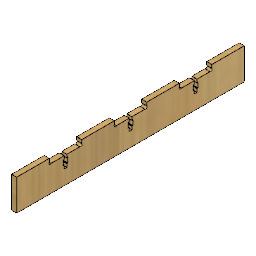
Bottom-plate-IIIS-square-rev1-40mm_8mm v1 (Autodesk Fusion 360 design; units mm, degrees)
Autodesk Fusion 360 part; units mm, degrees
sketch "Basic shape" plane through (0, 0, 0) normal (1, 0, 0) x (0, 0, -1)
  line L0 (0, 0) -> (-348.5, 0)
  line L1 (-348.5, 0) -> (-348.5, -48)
  line L2 (-348.5, -48) -> (0, -48)
  line L3 (0, -48) -> (0, 0)
  line L4 (-50, 0) -> (-99.5, 0)
  line L5 (-99.5, 0) -> (-99.5, -8)
  line L6 (-99.5, -8) -> (-50, -8)
  line L7 (-50, -8) -> (-50, 0)
  line L8 (-149.5, 0) -> (-199, 0)
  line L9 (-199, 0) -> (-199, -8)
  line L10 (-199, -8) -> (-149.5, -8)
  line L11 (-149.5, -8) -> (-149.5, 0)
  line L12 (-249, 0) -> (-298.5, 0)
  line L13 (-298.5, 0) -> (-298.5, -8)
  line L14 (-298.5, -8) -> (-249, -8)
  line L15 (-249, -8) -> (-249, 0)
  line L16 (-298.5, -8) -> (-348.5, -8) construction
  line L17 (-199, -8) -> (-249, -8) construction
  line L18 (-99.5, -8) -> (-149.5, -8) construction
  line L19 (-50, -8) -> (0, -8) construction
  dimension "d10" = 50
  dimension "d12" = 8
  dimension "d13" = 348.5
  dimension "d14" = 36.1667
  dimension "d246" = 40
  measures "d13" distance of L0.start
extrude "Extrude1" add sketch "Basic shape" along normal blind 8 contours L0 L1 L2 L3 L5 L6 L7 L9 L10 L11 L13 L14 L15
sketch "T slots" plane through (0, 0, 0) normal (-1, 0, 0) x (0, 0, 1)
  line L0 (348.5, 0) -> (298.5, 0)
  line L1 (298.5, 0) -> (298.5, -8)
  line L2 (298.5, -8) -> (249, -8)
  line L3 (249, -8) -> (249, 0)
  line L4 (249, 0) -> (199, 0)
  line L5 (199, 0) -> (199, -8)
  line L6 (199, -8) -> (149.5, -8)
  line L7 (149.5, -8) -> (149.5, 0)
  line L8 (149.5, 0) -> (99.5, 0)
  line L9 (99.5, 0) -> (99.5, -8)
  line L10 (99.5, -8) -> (50, -8)
  line L11 (50, -8) -> (50, 0)
  line L12 (50, 0) -> (0, 0)
  line L13 (0, 0) -> (0, -48)
  line L14 (0, -48) -> (348.5, -48)
  line L15 (348.5, -48) -> (348.5, 0)
  line L16 (72.74, -8) -> (76.76, -8)
  line L17 (76.76, -8) -> (76.76, -25.5)
  line L18 (76.76, -25.5) -> (72.74, -25.5)
  line L19 (72.74, -25.5) -> (72.74, -8)
  line L20 (71.27, -13) -> (78.27, -13)
  line L21 (78.27, -13) -> (78.27, -20.5)
  line L22 (78.27, -20.5) -> (71.27, -20.5)
  line L23 (71.27, -20.5) -> (71.27, -13)
  line L24 (170.77, -20.5) -> (170.77, -13)
  line L25 (172.24, -8) -> (176.26, -8)
  line L26 (170.77, -13) -> (177.77, -13)
  line L27 (172.24, -25.5) -> (172.24, -8)
  line L28 (176.26, -8) -> (176.26, -25.5)
  line L29 (177.77, -20.5) -> (170.77, -20.5)
  line L30 (177.77, -13) -> (177.77, -20.5)
  line L31 (176.26, -25.5) -> (172.24, -25.5)
  line L32 (277.27, -20.5) -> (270.27, -20.5)
  line L33 (270.27, -13) -> (277.27, -13)
  line L34 (275.76, -8) -> (275.76, -25.5)
  line L35 (271.74, -25.5) -> (271.74, -8)
  line L36 (275.76, -25.5) -> (271.74, -25.5)
  line L37 (271.74, -8) -> (275.76, -8)
  line L38 (277.27, -13) -> (277.27, -20.5)
  line L39 (270.27, -20.5) -> (270.27, -13)
  circle A0 centre (275.27, -15) radius 2
  circle A1 centre (275.27, -18.5) radius 2
  dimension "d17" = 17.5
  dimension "d18" = 4.02
  dimension "d19" = 7
  dimension "d20" = 1.51
  dimension "d21" = 5
  dimension "d23" = 7.5
  dimension "d29" = 2.01
  dimension "d247" = 17.5
  dimension "d248" = 4.02
  dimension "d249" = 7
  dimension "d250" = 1.51
  dimension "d251" = 5
  dimension "d252" = 7.5
  dimension "d253" = 2.01
  dimension "d254" = 17.5
  dimension "d255" = 4.02
  dimension "d256" = 7
  dimension "d257" = 1.51
  dimension "d258" = 5
  dimension "d259" = 7.5
  dimension "d260" = 2.01
  dimension "d357" = 4
  dimension "d358" = 4
  measures "d17" distance of L12.end
  measures "d20" distance of L17
  measures "d21" distance of L20
  measures "d23" distance of L12.end
  measures "d247" distance of L12.end
  measures "d250" distance of L28
  measures "d251" distance of L26
  measures "d252" distance of L12.end
  measures "d254" distance of L12.end
  measures "d257" distance of L34
  measures "d258" distance of L33
  measures "d259" distance of L12.end
  measures "d357" diameter of A0
  measures "d358" diameter of A1
extrude "Extrude2" cut sketch "T slots" against normal through all contours L2 L33 L34 L35 L37 | L33 L34 A0 | L33 L34 L38 A0 | L32 L33 L35 L39 | L32 L33 L35 A0 A1 | L34 A0 A1 | L34 A0 A1 | L32 L34 L35 L36 | L34 A0 A1 | L34 A0 A1 | L38 A0 A1 | L34 A0 A1 | L10 L16 L17 L19 L20 | L32 L34 A1 | L34 A0 A1 | L32 L34 L38 A1 | L17 L19 L20 L22 | L19 L20 L22 L23 | L17 L20 L21 L22 | L17 L18 L19 L22 | L6 L25 L26 L27 L28 | L26 L27 L28 L29 | L26 L28 L29 L30 | L24 L26 L27 L29 | L27 L28 L29 L31
hole "Hole24" at (8, -6.5858, 297.0858) direction (-1, 0, 0) diameter 4 end up to surface (8 mm away)
hole "Hole25" at (8, -6.5858, 51.4142) direction (-1, 0, 0) diameter 4 end up to surface (8 mm away)
hole "Hole26" at (8, -6.5858, 98.0858) direction (-1, 0, 0) diameter 4 end up to surface (8 mm away)
hole "Hole27" at (8, -6.5858, 197.5858) direction (-1, 0, 0) diameter 4 end up to surface (8 mm away)
hole "Hole28" at (8, -6.5858, 250.4142) direction (-1, 0, 0) diameter 4 end up to surface (8 mm away)
hole "Hole29" at (8, -6.5858, 150.9142) direction (-1, 0, 0) diameter 4 end up to surface (8 mm away)
equation "d10 = Square_joint_thickness"
equation "pannel_thickness = 8 mm"
equation "d12 = pannel_thickness * 3 / 3"
equation "d15 = pannel_thickness"
equation "d20 = ( ( ( 7 - 4 ) / 2 ) * 1 mm ) + 0.01 mm"
equation "d250 = ( ( ( 7 - 4 ) / 2 ) * 1 mm ) + 0.01 mm"
equation "d257 = ( ( ( 7 - 4 ) / 2 ) * 1 mm ) + 0.01 mm"
equation "dbToolDia = 4 mm"
equation "dbOffset = 0 mm" comment "Do NOT change formula"
equation "dbRadius = ( dbToolDia + dbOffset ) / 2" comment "Do NOT change formula"
equation "dbMinPercent = 10"
equation "dbHoleOffset = dbRadius / sqrt(2)" comment "Do NOT change formula"
equation "d530 = dbRadius * 2"
equation "d532 = dbHoleOffset"
equation "d533 = dbHoleOffset"
equation "d535 = dbRadius * 2"
equation "d537 = dbHoleOffset"
equation "d538 = dbHoleOffset"
equation "d540 = dbRadius * 2"
equation "d542 = dbHoleOffset"
equation "d543 = dbHoleOffset"
equation "d545 = dbRadius * 2"
equation "d547 = dbHoleOffset"
equation "d548 = dbHoleOffset"
equation "d550 = dbRadius * 2"
equation "d552 = dbHoleOffset"
equation "d553 = dbHoleOffset"
equation "d555 = dbRadius * 2"
equation "d557 = dbHoleOffset"
equation "d558 = dbHoleOffset"
equation "Square_joint_thickness = 50 mm"
